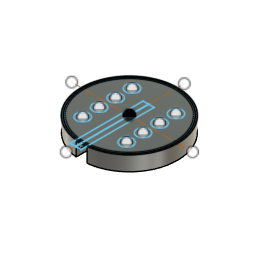
灯盘 v1 (Autodesk Fusion 360 design; units mm, degrees)
Autodesk Fusion 360 part; units mm, degrees
sketch "Sketch1" plane through (0, 0, 0) normal (0, 0, 1) x (1, 0, 0)
  circle A0 centre (0, 0) radius 16.5
  circle A1 centre (0, 0) radius 17.5
  circle A2 centre (0, 0) radius 17
  line L0 (0, 7) -> (2, 7)
  line L1 (2, 7) -> (2, -19.5649)
  line L2 (2, -19.5649) -> (0, -19.5649)
  line L3 (0, -19.5649) -> (0, 7)
  line L4 (0, 7) -> (-2, 7)
  line L5 (-2, 7) -> (-2, -19.5649)
  line L6 (-2, -19.5649) -> (0, -19.5649)
  line L7 (0, -19.5649) -> (0, 7)
  circle A3 centre (-8, 9) radius 2.2361
  circle A4 centre (-8, 3) radius 2.2361
  line L8 (-21, 0) -> (23, 0) construction
  circle A5 centre (-8, -9) radius 2.2361
  circle A6 centre (-8, -3) radius 2.2361
  line L9 (0, 20) -> (0, -23) construction
  circle A7 centre (8, 9) radius 2.2361
  circle A8 centre (8, 3) radius 2.2361
  circle A9 centre (8, -3) radius 2.2361
  circle A10 centre (8, -9) radius 2.2361
  dimension "d1" = 33
  dimension "d2" = 35
  dimension "d3" = 34
  dimension "d8" = 2
  dimension "d11" = 0
  dimension "d12" = -6
  constraint coincident A0.centre A1.centre
  constraint concentric A0 A1
  constraint concentric A0 A2
  constraint horizontal L0
  constraint vertical L1
  constraint horizontal L2
  constraint vertical L3
  constraint symmetric L0.start L3 L4.start
  constraint symmetric L0.end L3 L4.end
  constraint symmetric L1.end L3 L5.end
  constraint symmetric L2.end L3 L6.end
  constraint horizontal L8
  constraint symmetric A3 L8 A5
  constraint symmetric A4 L8 A6
  constraint vertical L9
  constraint symmetric A3 L9 A7
  constraint symmetric A4 L9 A8
  constraint symmetric A5 L9 A10
  constraint symmetric A6 L9 A9
  measures "d1" diameter of A0
  measures "d2" diameter of A1
  measures "d3" diameter of A2
  measures "d8" distance of L0.start L0.end
extrude "Extrude1" add sketch "Sketch1" against normal blind 5.4 contours A0 L0 L1 L4 L5 | A0 A2 L1 L5 | A0 L3 L4 L5 L7 | A0 A2 L3 L5 L7 | A0 A2 L1 L3 L7 | A0 L0 L1 L3 L7 | A1 A2 L1 L5 | A1 A2 L3 L5 L7 | A1 A2 L1 L3 L7 | A3 | A4 | A5 | A6 | A7 | A8 | A9 | A10 makes body 1
extrude "Extrude2" cut sketch "Sketch1" against normal blind 3.5 contours A0 L0 L1 L4 L5 | A0 L3 L4 L5 L7 | A0 A2 L3 L5 L7 | A0 A2 L1 L3 L7 | A0 L0 L1 L3 L7 | A3 | A4 | A5 | A6 | A7 | A8 | A9 | A10 bodies 1
extrude "Extrude3" cut sketch "Sketch1" against normal blind 10 contours A0 L3 L4 L5 L7 | A0 A2 L3 L5 L7 | A0 A2 L1 L3 L7 | A0 L0 L1 L3 L7 | A1 A2 L3 L5 L7 | A1 A2 L1 L3 L7 | A1 L3 L5 L6 L7 | A1 L1 L2 L3 L7 | A3 | A4 | A5 | A6 | A7 | A8 | A9 | A10 bodies 1
extrude "Extrude4" cut sketch "Sketch1" against normal blind 1 contours A0 A2 L1 L5 bodies 1
extrude "Extrude5" add sketch "Sketch1" against normal blind 0.6 separate body contours A0 L0 L1 L4 L5 | A0 A2 L1 L5 | A0 L3 L4 L5 L7 | A0 A2 L3 L5 L7 | A0 A2 L1 L3 L7 | A0 L0 L1 L3 L7 | A3 | A4 | A5 | A6 | A7 | A8 | A9 | A10 makes body 2
